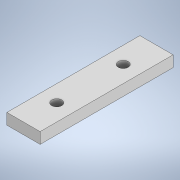
# Autodesk Inventor part: Ajuste vertical
Saved by Autodesk Inventor 2022 (Build 260153000, 153)
## iProperties
Created: 2022-02-28
Part Number: Ajuste vertical
Material: Generic
Document SubType Name: Modeling
Designer: hurta
Density: 1 g/cm^3
Appearance: Default
Author: hurta
Autodesk Inventor part; units mm, degrees
ref_plane "YZ Plane" through (0, 0, 0) normal (1, 0, 0) x (0, 1, 0)
ref_plane "XZ Plane" through (0, 0, 0) normal (0, 1, 0) x (-1, 0, 0)
ref_plane "XY Plane" through (0, 0, 0) normal (0, 0, 1) x (1, 0, 0)
sketch "Sketch1" plane through (0, 0, 0) normal (0, 1, 0) x (-1, 0, 0)
  line L0 (-7.5, -30) -> (7.5, -30)
  line L1 (7.5, -30) -> (7.5, 30)
  line L2 (7.5, 30) -> (-7.5, 30)
  line L3 (-7.5, 30) -> (-7.5, -30)
  line L4 (-7.5, -30) -> (7.5, 30) construction
  line L5 (7.5, -30) -> (-7.5, 30) construction
  point P0 (0, 0)
  dimension "d0" = 15
  dimension "d1" = 60
  constraints: 12 end point, 2 midpoint, 2 parallel, 1 horizontal, 1 perpendicular
  measures "d0" distance of L2.end L1.end
  measures "d1" distance of L1.end L0.end
extrude "Extrusion1" add sketch "Sketch1" along normal blind 5
sketch "Sketch2" plane through (0, 5, 0) normal (0, 1, 0) x (1, 0, 0)
  line L0 (-7.5, -30) -> (7.5, -30) projected
  line L1 (7.5, 30) -> (-7.5, 30) projected
  point P0 (0, 0)
  point P1 (0, -15)
  point P2 (0, 15)
  point P3 (0, -30)
  dimension "d4" = 15
  dimension "d5" = 15
  constraints: 2 vertical alignment, 1 midpoint
  measures "d4" distance from line of point (0, -15) L0
  measures "d5" distance from line of L1 point (0, 15)
hole "Hole1" at (0, 5, 15) at (0, 5, -15) direction (0, -1, 0) diameter 4.5 end through all
body "Solid1"
